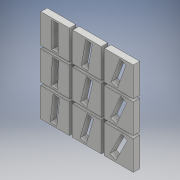
# Autodesk Inventor part: magnet-54-offset-27
Saved by Autodesk Inventor 2018 (Build 220112000, 112)
## iProperties
Created: 2025-03-17
Part Number: magnet-54-offset-27
Material: Generic
Document SubType Name: Modeling
Designer: neo
Density: 1 g/cm^3
Appearance: Default
Author: neo
Autodesk Inventor part; units mm, degrees
ref_plane "YZ Plane" through (0, 0, 0) normal (1, 0, 0) x (0, 1, 0)
ref_plane "XZ Plane" through (0, 0, 0) normal (0, 1, 0) x (-1, 0, 0)
ref_plane "XY Plane" through (0, 0, 0) normal (0, 0, 1) x (1, 0, 0)
sketch "Sketch1" plane through (0, 0, 0) normal (0, 1, 0) x (-1, 0, 0)
  line L0 (44.286, 57.5056) -> (-1.714, 57.5056)
  line L1 (-1.714, 57.5056) -> (-1.714, 11.5056)
  line L2 (-1.714, 11.5056) -> (44.286, 11.5056)
  line L3 (44.286, 11.5056) -> (44.286, 57.5056)
  line L4 (21.286, 57.5056) -> (21.286, 11.5056) construction
  line L5 (44.286, 34.5056) -> (-1.714, 34.5056) construction
  line L6 (12.4685, 52.0626) -> (21.286, 34.5056) construction
  line L7 (21.286, 34.5056) -> (12.2118, 29.9484) construction
  line L8 (16.8449, 54.8236) -> (7.6405, 50.201)
  line L9 (7.6405, 50.201) -> (25.7271, 14.1876)
  line L10 (25.7271, 14.1876) -> (34.9315, 18.8102)
  line L11 (34.9315, 18.8102) -> (16.8449, 54.8236)
  line L12 (94.286, 57.5056) -> (48.286, 57.5056)
  line L13 (48.286, 57.5056) -> (48.286, 11.5056)
  line L14 (48.286, 11.5056) -> (94.286, 11.5056)
  line L15 (94.286, 11.5056) -> (94.286, 57.5056)
  line L16 (71.286, 57.5056) -> (71.286, 11.5056) construction
  line L17 (94.286, 34.5056) -> (48.286, 34.5056) construction
  line L18 (65.6512, 53.327) -> (71.286, 34.5056) construction
  line L19 (71.286, 34.5056) -> (61.5583, 31.5933) construction
  line L20 (70.4406, 55.2861) -> (60.5733, 52.332)
  line L21 (60.5733, 52.332) -> (72.1314, 13.725)
  line L22 (72.1314, 13.725) -> (81.9987, 16.6791)
  line L23 (81.9987, 16.6791) -> (70.4406, 55.2861)
  line L24 (144.286, 57.5056) -> (98.286, 57.5056)
  line L25 (98.286, 57.5056) -> (98.286, 11.5056)
  line L26 (98.286, 11.5056) -> (144.286, 11.5056)
  line L27 (144.286, 11.5056) -> (144.286, 57.5056)
  line L28 (121.286, 57.5056) -> (121.286, 11.5056) construction
  line L29 (144.286, 34.5056) -> (98.286, 34.5056) construction
  line L30 (119.0051, 54.0195) -> (121.286, 34.5056) construction
  line L31 (121.286, 34.5056) -> (111.2004, 33.3267) construction
  line L32 (124.0619, 55.1172) -> (113.8315, 53.9214)
  line L33 (113.8315, 53.9214) -> (118.5101, 13.8939)
  line L34 (118.5101, 13.8939) -> (128.7404, 15.0897)
  line L35 (128.7404, 15.0897) -> (124.0619, 55.1172)
  line L36 (44.286, 107.5056) -> (-1.714, 107.5056)
  line L37 (-1.714, 107.5056) -> (-1.714, 61.5056)
  line L38 (-1.714, 61.5056) -> (44.286, 61.5056)
  line L39 (44.286, 61.5056) -> (44.286, 107.5056)
  line L40 (21.286, 107.5056) -> (21.286, 61.5056) construction
  line L41 (44.286, 84.5056) -> (-1.714, 84.5056) construction
  line L42 (13.5043, 102.5456) -> (21.286, 84.5056) construction
  line L43 (21.286, 84.5056) -> (11.9622, 80.4837) construction
  line L44 (18.0338, 105.0474) -> (8.5762, 100.9678)
  line L45 (8.5762, 100.9678) -> (24.5382, 63.9637)
  line L46 (24.5382, 63.9637) -> (33.9958, 68.0433)
  line L47 (33.9958, 68.0433) -> (18.0338, 105.0474)
  line L48 (44.286, 157.5056) -> (-1.714, 157.5056)
  line L49 (-1.714, 157.5056) -> (-1.714, 111.5056)
  line L50 (-1.714, 111.5056) -> (44.286, 111.5056)
  line L51 (44.286, 111.5056) -> (44.286, 157.5056)
  line L52 (21.286, 157.5056) -> (21.286, 111.5056) construction
  line L53 (44.286, 134.5056) -> (-1.714, 134.5056) construction
  line L54 (14.5664, 152.9675) -> (21.286, 134.5056) construction
  line L55 (21.286, 134.5056) -> (11.7441, 131.0326) construction
  line L56 (19.2337, 155.2018) -> (9.5549, 151.679)
  line L57 (9.5549, 151.679) -> (23.3383, 113.8094)
  line L58 (23.3383, 113.8094) -> (33.0171, 117.3322)
  line L59 (33.0171, 117.3322) -> (19.2337, 155.2018)
  line L60 (94.286, 107.5056) -> (48.286, 107.5056)
  line L61 (48.286, 107.5056) -> (48.286, 61.5056)
  line L62 (48.286, 61.5056) -> (94.286, 61.5056)
  line L63 (94.286, 61.5056) -> (94.286, 107.5056)
  line L64 (71.286, 107.5056) -> (71.286, 61.5056) construction
  line L65 (94.286, 84.5056) -> (48.286, 84.5056) construction
  line L66 (66.7551, 103.6228) -> (71.286, 84.5056) construction
  line L67 (71.286, 84.5056) -> (61.4055, 82.1638) construction
  line L68 (71.6503, 105.3001) -> (61.6279, 102.9248)
  line L69 (61.6279, 102.9248) -> (70.9217, 63.711)
  line L70 (70.9217, 63.711) -> (80.9441, 66.0864)
  line L71 (80.9441, 66.0864) -> (71.6503, 105.3001)
  line L72 (94.286, 157.5056) -> (48.286, 157.5056)
  line L73 (48.286, 157.5056) -> (48.286, 111.5056)
  line L74 (48.286, 111.5056) -> (94.286, 111.5056)
  line L75 (94.286, 111.5056) -> (94.286, 157.5056)
  line L76 (71.286, 157.5056) -> (71.286, 111.5056) construction
  line L77 (94.286, 134.5056) -> (48.286, 134.5056) construction
  line L78 (67.8744, 153.8539) -> (71.286, 134.5056) construction
  line L79 (71.286, 134.5056) -> (61.286, 132.7423) construction
  line L80 (72.8587, 155.2437) -> (62.7152, 153.4552)
  line L81 (62.7152, 153.4552) -> (69.7132, 113.7674)
  line L82 (69.7132, 113.7674) -> (79.8568, 115.556)
  line L83 (79.8568, 115.556) -> (72.8587, 155.2437)
  line L84 (144.286, 107.5056) -> (98.286, 107.5056)
  line L85 (98.286, 107.5056) -> (98.286, 61.5056)
  line L86 (98.286, 61.5056) -> (144.286, 61.5056)
  line L87 (144.286, 61.5056) -> (144.286, 107.5056)
  line L88 (121.286, 107.5056) -> (121.286, 61.5056) construction
  line L89 (144.286, 84.5056) -> (98.286, 84.5056) construction
  line L90 (120.1436, 104.1191) -> (121.286, 84.5056) construction
  line L91 (121.286, 84.5056) -> (111.1489, 83.9152) construction
  line L92 (125.2557, 104.9209) -> (114.9731, 104.322)
  line L93 (114.9731, 104.322) -> (117.3163, 64.0902)
  line L94 (117.3163, 64.0902) -> (127.5989, 64.6891)
  line L95 (127.5989, 64.6891) -> (125.2557, 104.9209)
  line L96 (144.286, 157.5056) -> (98.286, 157.5056)
  line L97 (98.286, 157.5056) -> (98.286, 111.5056)
  line L98 (98.286, 111.5056) -> (144.286, 111.5056)
  line L99 (144.286, 111.5056) -> (144.286, 157.5056)
  line L100 (121.286, 157.5056) -> (121.286, 111.5056) construction
  line L101 (144.286, 134.5056) -> (98.286, 134.5056) construction
  line L102 (121.286, 154.1524) -> (121.286, 134.5056) construction
  line L103 (121.286, 134.5056) -> (111.1318, 134.5056) construction
  line L104 (126.436, 154.6556) -> (116.136, 154.6556)
  line L105 (116.136, 154.6556) -> (116.136, 114.3556)
  line L106 (116.136, 114.3556) -> (126.436, 114.3556)
  line L107 (126.436, 114.3556) -> (126.436, 154.6556)
  dimension "w" = 46
  dimension "d65" = 46
  dimension "d" = 10.3
  dimension "d67" = 40.3
  dimension "d68" = 116.667
  dimension "d69" = 46
  dimension "d70" = 46
  dimension "d71" = 10.3
  dimension "d72" = 40.3
  dimension "d73" = 106.667
  dimension "d76" = 46
  dimension "d77" = 46
  dimension "d78" = 10.3
  dimension "d79" = 40.3
  dimension "d80" = 96.667
  dimension "d83" = 46
  dimension "d84" = 46
  dimension "d85" = 10.3
  dimension "d86" = 40.3
  dimension "d87" = 113.333
  dimension "d90" = 46
  dimension "d91" = 46
  dimension "d92" = 10.3
  dimension "d93" = 40.3
  dimension "d94" = 110
  dimension "d97" = 46
  dimension "d98" = 46
  dimension "d99" = 10.3
  dimension "d100" = 40.3
  dimension "d101" = 103.333
  dimension "d104" = 46
  dimension "d105" = 46
  dimension "d106" = 10.3
  dimension "d107" = 40.3
  dimension "d108" = 100
  dimension "d111" = 46
  dimension "d112" = 46
  dimension "d113" = 10.3
  dimension "d114" = 40.3
  dimension "d115" = 93.333
  dimension "d118" = 46
  dimension "d119" = 46
  dimension "d120" = 10.3
  dimension "d121" = 40.3
  dimension "d122" = 90
  constraints: 216 end point, 45 midpoint, 36 perpendicular, 18 equal length, 18 parallel, 9 horizontal, 18 other
  measures "w" distance of L2.end L0.start
  measures "d65" distance of L0.start L0.end
  measures "d" distance between parallel lines of L9 L11
  measures "d67" distance between parallel lines of L10 L8
  measures "d68" angle of L5 L6
  measures "d69" distance of L14.end L12.start
  measures "d70" distance of L12.start L12.end
  measures "d71" distance between parallel lines of L21 L23
  measures "d72" distance between parallel lines of L22 L20
  measures "d73" angle of L17 L18
  measures "d76" distance of L26.end L24.start
  measures "d77" distance of L24.start L24.end
  measures "d78" distance between parallel lines of L33 L35
  measures "d79" distance between parallel lines of L34 L32
  measures "d80" angle of L29 L30
  measures "d83" distance of L38.end L36.start
  measures "d84" distance of L36.start L36.end
  measures "d85" distance between parallel lines of L45 L47
  measures "d86" distance between parallel lines of L46 L44
  measures "d87" angle of L41 L42
  measures "d90" distance of L50.end L48.start
  measures "d91" distance of L48.start L48.end
  measures "d92" distance between parallel lines of L57 L59
  measures "d93" distance between parallel lines of L58 L56
  measures "d94" angle of L53 L54
  measures "d97" distance of L62.end L60.start
  measures "d98" distance of L60.start L60.end
  measures "d99" distance between parallel lines of L69 L71
  measures "d100" distance between parallel lines of L70 L68
  measures "d101" angle of L65 L66
  measures "d104" distance of L74.end L72.start
  measures "d105" distance of L72.start L72.end
  measures "d106" distance between parallel lines of L81 L83
  measures "d107" distance between parallel lines of L82 L80
  measures "d108" angle of L77 L78
  measures "d111" distance of L86.end L84.start
  measures "d112" distance of L84.start L84.end
  measures "d113" distance between parallel lines of L93 L95
  measures "d114" distance between parallel lines of L94 L92
  measures "d115" angle of L89 L90
  measures "d118" distance of L98.end L96.start
  measures "d119" distance of L96.start L96.end
  measures "d120" distance between parallel lines of L105 L107
  measures "d121" distance between parallel lines of L106 L104
  measures "d122" angle of L101 L102
extrude "Extrusion1" add sketch "Sketch1" along normal blind 10
chamfer "Chamfer1" distance 1 angle 45 18 edges at (-144.286, 10, 134.5056) (-144.286, 10, 84.5056) (-144.286, 10, 34.5056) (-94.286, 10, 134.5056) (-94.286, 10, 84.5056) (-94.286, 10, 34.5056) (-44.286, 10, 34.5056) (-44.286, 10, 84.5056) (-44.286, 10, 134.5056) (-144.286, 5, 157.5056) (-144.286, 5, 107.5056) (-144.286, 5, 57.5056) (-94.286, 5, 157.5056) (-94.286, 5, 107.5056) (-94.286, 5, 57.5056) (-44.286, 5, 157.5056) (-44.286, 5, 107.5056) (-44.286, 5, 57.5056)
equation "\"d68\" = a0 + 8 * ad"
equation "\"d73\" = a0 + 5 * ad"
equation "\"d80\" = a0 + 2 * ad"
equation "\"d87\" = a0 + 7 * ad"
equation "\"d94\" = a0 + 6 * ad"
equation "\"d101\" = a0 + 4 * ad"
equation "\"d108\" = a0 + 3 * ad"
equation "\"d115\" = a0 + ad"
equation "\"d122\" = a0 + 0 * ad"
equation "\"ad\" = 3.33333deg"
equation "\"d74\" = 0 * d75"
equation "\"d75\" = 3.333333deg"
equation "\"d81\" = 0 * d82"
equation "\"d82\" = 3.333333deg"
equation "\"d88\" = 0 * d89"
equation "\"d89\" = 3.333333deg"
equation "\"d95\" = 0 * d96"
equation "\"d96\" = 3.333333deg"
equation "\"d102\" = 0 * d103"
equation "\"d103\" = 3.333333deg"
equation "\"d109\" = 0 * d110"
equation "\"d110\" = 3.333333deg"
equation "\"d116\" = 0 * d117"
equation "\"d117\" = 3.333333deg"
equation "\"d123\" = 0 * d124"
equation "\"d124\" = 3.333333deg"
equation "\"a0\" = 90deg"
body "Solid1"
